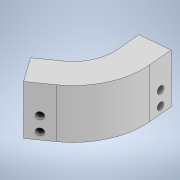
# Autodesk Inventor part: Soporte
Saved by Autodesk Inventor 2021 (Build 250183000, 183)
## iProperties
Created: 2023-12-04
Part Number: Soporte
Material: Generic
Document SubType Name: Modeling
Designer: Nicol
Density: 1 g/cm^3
Appearance: Default
Author: Nicol
Autodesk Inventor part; units mm, degrees
ref_plane "YZ Plane" through (0, 0, 0) normal (1, 0, 0) x (0, 1, 0)
ref_plane "XZ Plane" through (0, 0, 0) normal (0, 1, 0) x (-1, 0, 0)
ref_plane "XY Plane" through (0, 0, 0) normal (0, 0, 1) x (1, 0, 0)
sketch "Sketch1" plane through (0, 0, 0) normal (0, 1, 0) x (-1, 0, 0)
  arc A0 (7.3141, 15.8982) -> (0, 0) centre (17.4253, 1.6149) ccw
  arc A1 (0.0437, 26.1686) -> (-12.541, -1.0355) centre (17.4253, 1.6149) ccw
  line L0 (7.3141, 15.8982) -> (0.0437, 26.1686)
  line L1 (7.3141, 15.8982) -> (15.476, 21.6761)
  line L2 (0.0437, 26.1686) -> (9.8323, 33.098)
  line L3 (15.476, 21.6761) -> (8.2056, 31.9464)
  line L4 (11.395, 18.7872) -> (4.1246, 29.0575)
  line L5 (0, 0) -> (0.4614, -4.9787)
  line L6 (0.4614, -4.9787) -> (-12.0679, -6.1398)
  line L7 (-12.0679, -6.1398) -> (-12.541, -1.0355)
  line L8 (0.4614, -4.9787) -> (0.9228, -9.9573)
  line L9 (0.9228, -9.9573) -> (-11.6065, -11.1185)
  line L10 (-12.0679, -6.1398) -> (-11.6065, -11.1185)
  dimension "d3" = 10
  dimension "d5" = 12.5833
  dimension "d6" = 12.5833
  dimension "d8" = 17.5
  dimension "d9" = 5
  dimension "d11" = 5
  dimension "d12" = 12.583
  dimension "d13" = 60
  dimension "d14" = 90
  dimension "d16" = 90
  dimension "d17" = 5
  constraints: 22 end point, 4 point on circle, 3 tangent, 2 centre point, 1 parallel, 1 perpendicular, 1 point on line
  measures "d3" distance of L0.start L1.end
  measures "d5" distance of L0.start L0.end
  measures "d6" distance of L1.end L3.end
  measures "d8" radius of A0
  measures "d9" distance between parallel lines of L0 L4
  measures "d11" distance of L5.start L5.end
  measures "d12" distance of L5.end L6.end
  measures "d13" angle of L4 L6
  measures "d14" angle of L5 L6
  measures "d16" angle of L6 L7
  measures "d17" distance of L5.end L8.end
extrude "Extrusion1" add sketch "Sketch1" along normal blind 21
sketch "Sketch2" plane through (0, 0, 0) normal (-0.9957, 0, 0.0923) x (0.0923, 0, 0.9957)
  circle A0 centre (-5, 9) radius 1.5
  line L0 (-10, 0) -> (0, 0) projected
  circle A1 centre (-5, 3) radius 1.5
  line L1 (-10, 0) -> (-10, 21) projected
  dimension "d20" = 3
  dimension "d22" = 3
  dimension "d23" = 6
  dimension "d24" = 3
  dimension "d25" = 5
  dimension "d26" = 5
  constraints: 2 centre point
  measures "d20" diameter of A0
  measures "d22" diameter of A1
  measures "d23" distance of A0.centre A1.centre
  measures "d24" distance from line of L0 A1.centre
  measures "d25" distance from line of L1 A1.centre
  measures "d26" distance from line of L1 A0.centre
sketch "Sketch3" plane through (-15.476, 0, 21.6761) normal (-0.5778, 0, -0.8162) x (-0.8162, 0, 0.5778)
  circle A0 centre (-5, 3) radius 1.5
  circle A1 centre (-5, 9) radius 1.5
  line L0 (-10, 0) -> (0, 0) projected
  line L1 (0, 0) -> (0, 21) projected
  point P0 (-25.1554, 0)
  dimension "d27" = 3
  dimension "d28" = 3
  dimension "d29" = 6
  dimension "d30" = 0
  dimension "d31" = 3
  dimension "d32" = 5
  constraints: 2 centre point
  measures "d27" diameter of A0
  measures "d28" diameter of A1
  measures "d29" distance of A1.centre A0.centre
  measures "d30" horizontal distance of A0.centre A1.centre
  measures "d31" distance from line of L0 A0.centre
  measures "d32" distance from line of L1 A0.centre
extrude "Extrusion2" cut sketch "Sketch3" against normal blind 300
extrude "Extrusion3" cut sketch "Sketch2" against normal through all
body "Solid1"
